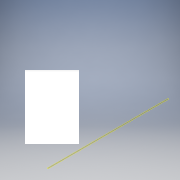
# Autodesk Inventor part: 04_Mirror
Saved by Autodesk Inventor 2016 (Build 200138000, 138)
## iProperties
Created: 2016-11-08
Part Number: 04_Mirror
Material: Generisch
Document SubType Name: Modeling
Designer: Bene
Density: 1 g/cm^3
Appearance: Chrom - poliert
Author: Bene
Autodesk Inventor part; units mm, degrees
ref_plane "YZ Plane" through (0, 0, 0) normal (1, 0, 0) x (0, 1, 0)
ref_plane "XZ Plane" through (0, 0, 0) normal (0, 1, 0) x (-1, 0, 0)
ref_plane "XY Plane" through (0, 0, 0) normal (0, 0, 1) x (1, 0, 0)
ref_plane "Arbeitsebene1" through (0, 141, -63) normal (0, 0, -1) x (-1, 0, 0)
sketch "Skizze1" plane through (0, 141, -63) normal (0, 0, -1) x (-1, 0, 0)
  line L0 (10.0029, -84.0029) -> (8.5887, -85.4171)
  line L1 (8.5887, -85.4171) -> (38.2872, -115.1156)
  line L2 (38.2872, -115.1156) -> (39.7014, -113.7014)
  line L3 (39.7014, -113.7014) -> (10.0029, -84.0029)
  line L4 (10.0029, -84.0029) -> (12.0029, -84.0029) construction
  line L5 (26, -77) -> (26, -127) projected
  line L6 (26, -100) -> (66, -100) projected
  point P0 (0, -141)
  dimension "d0" = 2
  dimension "d1" = 135
  dimension "d2" = 42
  constraints: 10 end point, 2 parallel, 1 equal length, 1 horizontal, 1 perpendicular, 1 point on line
  measures "d0" distance of L0.start L0.end
  measures "d1" angle of L0 L4
  measures "d2" distance of L1.end L0.end
extrude "Extrusion1" add sketch "Skizze1" along normal blind 3 and the other way blind 66
